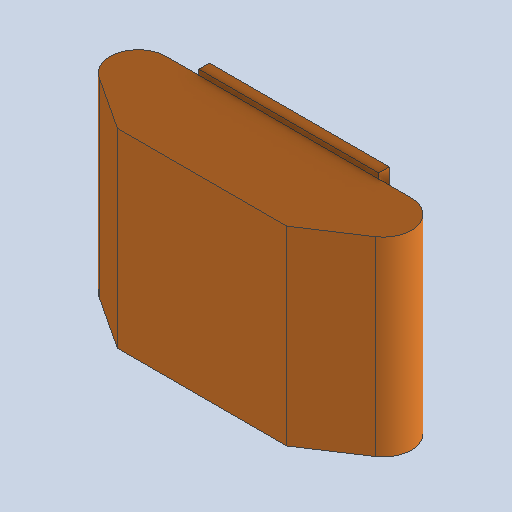
# Autodesk Inventor part: Roller platform
Saved by Autodesk Inventor 2025 (Build 290162010, 162A)
## iProperties
Created: 2024-07-02
Part Number: Roller platform
Material: Generic
Document SubType Name: Modeling
Designer: pokla
Density: 1 g/cm^3
Appearance: Default
Stock Number: Транспортно-роликовая платформа
Author: pokla
Autodesk Inventor part; units mm, degrees
ref_plane "YZ Plane" through (0, 0, 0) normal (1, 0, 0) x (0, 1, 0)
ref_plane "XZ Plane" through (0, 0, 0) normal (0, 1, 0) x (-1, 0, 0)
ref_plane "XY Plane" through (0, 0, 0) normal (0, 0, 1) x (1, 0, 0)
sketch "Sketch1" plane through (0, 0, 0) normal (0, 0, 1) x (1, 0, 0)
  line L0 (-142.5, 102) -> (142.5, 102) construction
  line L1 (142.5, 102) -> (142.5, 82) construction
  line L2 (142.5, 0) -> (-142.5, 0)
  line L3 (-142.5, 0) -> (-142.5, 82)
  line L4 (-142.5, 82) -> (142.5, 82)
  line L5 (142.5, 82) -> (142.5, 0)
  line L6 (80, 0) -> (142.5, 41)
  circle A0 centre (115.876, 55.376) radius 26.624
  line L7 (-142.5, 82) -> (-142.5, 102) construction
  line L8 (-80, 0) -> (-142.5, 41)
  circle A1 centre (-115.876, 55.376) radius 26.624
  point P0 (0, 0)
  point P1 (0, 0)
  point P2 (-130.4796, 33.1146)
  point P3 (130.4796, 33.1146)
  point P4 (115.876, 82)
  point P5 (-115.876, 82)
  dimension "d7" = 285
  dimension "d8" = 102
  dimension "d9" = 82
  dimension "d13" = 80
  dimension "d14" = 80
  constraints: 18 end point, 6 tangent, 5 parallel, 4 perpendicular, 3 midpoint, 2 centre point, 2 point on line, 1 coincident, 1 horizontal
  measures "d7" distance of L2.start L2.end
  measures "d8" distance of L0.end L2.start
  measures "d9" distance between parallel lines of L2 L4
  measures "d13" distance of L6.start point (0, 0)
  measures "d14" distance of point (0, 0) L8.start
extrude "Extrusion1" add sketch "Sketch1" along normal mid plane 180 contours L2 L8 A1 L4 A0 L6 | A0 | A1
sketch "Sketch2" plane through (-115.876, 82, 90) normal (0, 1, 0) x (1, 0, 0)
  line L0 (30.876, -5) -> (200.876, -5)
  line L1 (200.876, -5) -> (200.876, 185)
  line L2 (200.876, 185) -> (30.876, 185)
  line L3 (30.876, 185) -> (30.876, -5)
  line L4 (30.876, -5) -> (200.876, 185) construction
  point P0 (115.876, 90)
  point P1 (115.876, 90)
  dimension "d17" = 190
  dimension "d18" = 170
  constraints: 10 end point, 2 parallel, 1 coincident, 1 horizontal, 1 midpoint, 1 perpendicular
  measures "d17" distance of L0.end L1.end
  measures "d18" distance of L0.start L0.end
extrude "Extrusion2" add sketch "Sketch2" along normal blind 10
sketch "Sketch3" plane through (0, 0, 0) normal (0, 1, 0) x (-1, 0, 0)
  circle A0 centre (0, 0) radius 69
  dimension "d21" = 138
  constraints: 1 centre point, 1 coincident
  measures "d21" diameter of A0
extrude "Extrusion3" add sketch "Sketch3" along normal blind 102
equation "\"d14\" = d13"
body "Solid1"
